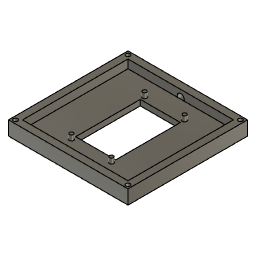
case top (Autodesk Fusion 360 design; units mm, degrees)
Autodesk Fusion 360 part; units mm, degrees
note: some values were not read from the file. Set by a fixed rule: which sketch regions a step uses.
sketch "Sketch1" plane through (0, 0, 0) normal (0, 0, 1) x (1, 0, 0)
  line L0 (0, 0) -> (0, 75)
  line L1 (0, 75) -> (75, 75)
  line L2 (0, 0) -> (75, 0)
  line L3 (75, 0) -> (75, 75)
  line L4 (75, 75) -> (0, 75)
  line L5 (0, 75) -> (0, 0)
  line L6 (-5, -5) -> (80, -5)
  line L7 (80, -5) -> (80, 80)
  line L8 (80, 80) -> (-5, 80)
  line L9 (-5, 80) -> (-5, -5)
  line L10 (-5, -5) -> (80, -5)
  line L11 (80, -5) -> (80, 80)
  dimension "d1" = 75
  dimension "d2" = 75
  dimension "d3" = 85
  constraint coincident L0.start L2.start
  constraint vertical L0
  constraint perpendicular L0 L1
  constraint horizontal L2
  constraint vertical L3
  constraint horizontal L4
  constraint vertical L5
  constraint horizontal L6
  constraint perpendicular L6 L7
  constraint horizontal L8
  constraint vertical L9
  constraint horizontal L10
  constraint vertical L11
  measures "d1" distance of L0.start L0.end
  measures "d2" distance of L0.end L1.end
  measures "d3" distance of L6.end L7.end
extrude "Extrude1" add sketch "Sketch1" along normal blind 10
sketch "Sketch2" plane through (0, 0, 0) normal (0, 0, 1) x (1, 0, 0)
  line L0 (0, 0) -> (75, 0)
  line L1 (75, 0) -> (75, 75)
  line L2 (75, 75) -> (0, 75)
  line L3 (0, 75) -> (0, 0)
  constraint horizontal L0
  constraint vertical L1
  constraint horizontal L2
  constraint vertical L3
  constraint coincident L0.start L3.end
extrude "Extrude2" add sketch "Sketch2" along normal blind 4
sketch "Sketch3" plane through (0, 0, 4) normal (0, 0, 1) x (-1, 0, 0)
  line L0 (0, -75) -> (0, 0)
  line L1 (0, 0) -> (-75, 0)
  line L2 (-75, 0) -> (-75, -75)
  line L3 (-75, -75) -> (0, -75)
  line L4 (0, -75) -> (-75, 0)
  line L5 (0, 0) -> (-75, -75)
  line L6 (-37.5, -37.5) -> (-20.25, -37.5)
  line L7 (-37.5, -37.5) -> (-54.75, -37.5)
  line L8 (-20.25, -37.5) -> (-20.25, -66.5)
  line L9 (-54.75, -37.5) -> (-54.75, -8.5)
  line L10 (-20.25, -66.5) -> (-54.75, -66.5)
  line L11 (-54.75, -66.5) -> (-54.75, -8.5)
  line L12 (-54.75, -8.5) -> (-20.25, -8.5)
  line L13 (-20.25, -8.5) -> (-20.25, -66.5)
  line L14 (-37.5, -37.5) -> (-37.5, -60.5)
  line L15 (-37.5, -37.5) -> (-37.5, -14.5)
  line L16 (-37.5, -14.5) -> (-51.75, -14.5)
  line L17 (-37.5, -60.5) -> (-23.25, -60.5)
  line L18 (-23.25, -60.5) -> (-51.75, -60.5)
  line L19 (-51.75, -60.5) -> (-51.75, -14.5)
  line L20 (-51.75, -14.5) -> (-23.25, -14.5)
  line L21 (-23.25, -14.5) -> (-23.25, -60.5)
  dimension "d8" = 17.25
  dimension "d9" = 17.25
  dimension "d10" = 29
  dimension "d11" = 29
  dimension "d12" = 23
  dimension "d13" = 23
  dimension "d14" = 14.25
  dimension "d15" = 14.25
  constraint coincident L0.start L3.end
  constraint coincident L1.end L2.start
  constraint coincident L0.end L1.start
  constraint coincident L2.end L3.start
  constraint midpoint L4 L6.start
  constraint parallel L3 L6
  constraint parallel L6 L7
  constraint perpendicular L6 L8
  constraint perpendicular L7 L9
  constraint horizontal L10
  constraint vertical L11
  constraint horizontal L12
  constraint vertical L13
  constraint perpendicular L6 L14
  constraint perpendicular L7 L15
  constraint perpendicular L15 L16
  constraint perpendicular L14 L17
  constraint horizontal L18
  constraint vertical L19
  constraint horizontal L20
  constraint vertical L21
  measures "d8" distance of L6.start L6.end
  measures "d9" distance of L6.start L7.end
  measures "d10" distance of L6.end L8.end
  measures "d11" distance of L7.end L9.end
  measures "d12" distance of L6.start L14.end
  measures "d13" distance of L6.start L15.end
  measures "d14" distance of L15.end L16.end
  measures "d15" distance of L14.end L17.end
extrude "Extrude3" cut sketch "Sketch3" against normal blind 5 contours L4 L14 L17 L18 L21 | L4 L6 L21 | L5 L6 L21 | L5 L15 L20 L21 | L5 L7 L19 | L5 L14 L18 L19 | L4 L7 L19 | L4 L15 L16 L19 L20
sketch "Sketch4" plane through (0, 0, 4) normal (0, 0, 1) x (-1, 0, 0)
  line L0 (-51.75, -60.5) -> (-51.75, -14.5)
  line L1 (-51.75, -14.5) -> (-23.25, -14.5)
  line L2 (-23.25, -14.5) -> (-23.25, -60.5)
  line L3 (-23.25, -60.5) -> (-51.75, -60.5)
  line L4 (0, -75) -> (0, 0)
  line L5 (0, 0) -> (-75, 0)
  line L6 (-75, 0) -> (-75, -75)
  line L7 (-75, -75) -> (0, -75)
  line L8 (-75, 0) -> (0, -75)
  line L9 (-75, -75) -> (0, 0)
  line L10 (-37.5, -37.5) -> (-54.75, -37.5)
  line L11 (-54.75, -37.5) -> (-54.75, -8.5)
  line L12 (-54.75, -8.5) -> (-20.25, -8.5)
  line L13 (-20.25, -8.5) -> (-20.25, -66.5)
  line L14 (-20.25, -66.5) -> (-54.75, -66.5)
  line L15 (-54.75, -66.5) -> (-54.75, -8.5)
  line L16 (-54.75, -8.5) -> (-20.25, -8.5)
  line L17 (-20.25, -8.5) -> (-20.25, -66.5)
  line L18 (-20.25, -66.5) -> (-20.25, -63.5)
  line L19 (-20.25, -63.5) -> (-23.25, -63.5)
  circle A0 centre (-23.25, -63.5) radius 1.6
  line L20 (-54.75, -66.5) -> (-51.75, -66.5)
  line L21 (-51.75, -66.5) -> (-51.75, -63.5)
  circle A1 centre (-51.75, -63.5) radius 1.6
  line L22 (-20.25, -8.5) -> (-23.25, -8.5)
  line L23 (-23.25, -8.5) -> (-23.25, -11.5)
  circle A2 centre (-23.25, -11.5) radius 1.6
  line L24 (-54.75, -8.5) -> (-54.75, -11.5)
  line L25 (-54.75, -11.5) -> (-51.75, -11.5)
  circle A3 centre (-51.75, -11.5) radius 1.6
  dimension "d23" = 17.25
  dimension "d24" = 29
  dimension "d25" = 34.5
  dimension "d26" = 58
  dimension "d27" = 3
  dimension "d28" = 3
  dimension "d29" = 3.2
  dimension "d30" = 3
  dimension "d31" = 3
  dimension "d32" = 3.2
  dimension "d33" = 3
  dimension "d34" = 3
  dimension "d35" = 3.2
  dimension "d36" = 3
  dimension "d37" = 3
  dimension "d38" = 3.2
  constraint coincident L5.end L6.start
  constraint coincident L4.start L7.end
  constraint coincident L6.end L7.start
  constraint coincident L4.end L5.start
  constraint midpoint L8 L10.start
  constraint parallel L5 L10
  constraint perpendicular L10 L11
  constraint perpendicular L11 L12
  constraint perpendicular L1 L13
  constraint horizontal L14
  constraint vertical L15
  constraint horizontal L16
  constraint vertical L17
  constraint perpendicular L14 L18
  constraint perpendicular L17 L19
  constraint coincident L19.end A0.centre
  constraint perpendicular L15 L20
  constraint perpendicular L20 L21
  constraint coincident L21.end A1.centre
  constraint perpendicular L17 L22
  constraint perpendicular L12 L23
  constraint coincident L23.end A2.centre
  constraint perpendicular L12 L24
  constraint perpendicular L24 L25
  constraint coincident L25.end A3.centre
  measures "d23" distance of L10.start L10.end
  measures "d24" distance of L10.end L11.end
  measures "d25" distance of L11.end L12.end
  measures "d26" distance of L12.end L13.end
  measures "d27" distance of L13.end L18.end
  measures "d28" distance of L18.end L19.end
  measures "d29" diameter of A0
  measures "d30" distance of L14.end L20.end
  measures "d31" distance of L20.end L21.end
  measures "d32" diameter of A1
  measures "d33" distance of L12.end L22.end
  measures "d34" distance of L22.end L23.end
  measures "d35" diameter of A2
  measures "d36" distance of L11.end L24.end
  measures "d37" distance of L24.end L25.end
  measures "d38" diameter of A3
extrude "Extrude4" add sketch "Sketch4" along normal blind 3.5 draft -4 contours A0 | A1 | A2 | A3
sketch "Sketch5" plane through (0, 0, 10) normal (0, 0, 1) x (-1, 0, 0)
  line L0 (0, 0) -> (0, -75)
  line L1 (0, -75) -> (-75, -75)
  line L2 (-75, -75) -> (-75, 0)
  line L3 (-75, 0) -> (0, 0)
  line L4 (-80, 5) -> (-80, -80)
  line L5 (-80, -80) -> (5, -80)
  line L6 (5, -80) -> (5, 5)
  line L7 (5, 5) -> (-80, 5)
  line L8 (5, 5) -> (0, 0)
  line L9 (5, 0) -> (0, 5)
  circle A0 centre (2.5, 2.5) radius 1.5
  line L10 (-75, 0) -> (-80, 5)
  circle A1 centre (-77.5, 2.5) radius 1.5
  line L11 (-75, 5) -> (-80, 0)
  circle A2 centre (-77.5, -77.5) radius 1.5
  circle A3 centre (2.5, -77.5) radius 1.5
  dimension "d41" = 3
  dimension "d43" = 3
  dimension "d44" = 3
  dimension "d45" = 3
  constraint coincident L6.end L7.start
  constraint coincident L0.start L3.end
  constraint coincident L6 L9.start
  constraint perpendicular L8 L9
  constraint midpoint L8 A0.centre
  constraint coincident L2.end L3.start
  constraint coincident L4.start L7.end
  constraint midpoint L10 A1.centre
  constraint coincident L7 L11.start
  constraint coincident L4 L11.end
  measures "d41" diameter of A0
  measures "d43" diameter of A1
  measures "d44" diameter of A2
  measures "d45" diameter of A3
extrude "Extrude5" cut sketch "Sketch5" against normal blind 4 contours L8 L9 A0 | L8 L9 A0 | L10 A1 L11 | L10 A1 L11 | L8 L9 A0 | L8 L9 A0 | L10 A1 L11 | L10 A1 L11 | A2 | A3
sketch "Sketch6" plane through (0, 75, 0) normal (0, -1, 0) x (1, 0, 0)
  line L0 (0, 4) -> (75, 4)
  line L1 (75, 4) -> (75, 10)
  line L2 (75, 10) -> (0, 10)
  line L3 (0, 10) -> (0, 4)
  line L4 (75, 4) -> (0, 10)
  line L5 (0, 4) -> (75, 10)
  line L6 (38.5, 6.7) -> (36.5, 6.7)
  line L7 (36.5, 6.7) -> (36.5, 7.3)
  line L8 (36.5, 7.3) -> (38.5, 7.3)
  line L9 (38.5, 7.3) -> (38.5, 6.7)
  line L10 (38.5, 6.7) -> (36.5, 7.3) construction
  line L11 (36.5, 6.7) -> (38.5, 7.3) construction
  point P0 (37.5, 7)
  constraint coincident L0.end L1.start
  constraint coincident L2.end L3.start
  constraint coincident L0.start L3.end
  constraint coincident L1.end L2.start
  constraint horizontal L6
  constraint perpendicular L6 L7
  constraint parallel L6 L8
  constraint parallel L7 L9
  constraint coincident L10 P0
  constraint coincident L11 P0
  constraint midpoint L4 P0
extrude "Extrude6" cut sketch "Sketch6" against normal blind 5 contours L4 L5 L7 | L4 L5 L6 L7 L9 | L4 L5 L9 | L4 L5 L7 L8 L9
sketch "Sketch7" plane through (0, 80, 0) normal (0, 1, 0) x (-1, 0, 0)
  line L0 (-36.5, 7.3) -> (-36.5, 6.7)
  line L1 (-38.5, 6.7) -> (-38.5, 7.3)
  line L2 (-80, 0) -> (5, 0)
  line L3 (5, 0) -> (5, 10)
  line L4 (5, 10) -> (-80, 10)
  line L5 (-80, 10) -> (-80, 0)
  line L6 (5, 0) -> (-80, 10)
  line L7 (-80, 0) -> (5, 10)
  circle A0 centre (-37.5, 5) radius 2.5
  dimension "d50" = 5
  constraint coincident L2.end L3.start
  constraint coincident L4.end L5.start
  constraint coincident L2.start L5.end
  constraint coincident L3.end L4.start
  constraint midpoint L6 A0.centre
  measures "d50" diameter of A0
extrude "Extrude7" cut sketch "Sketch7" against normal blind 5 contours L6 L7 A0 | L6 L7 A0 | L6 L7 A0 | L6 L7 A0
equation "d8 = ( 34.5 / 2 ) * 1 mm"
equation "d9 = ( 34.5 / 2 ) * 1 mm"
equation "d10 = ( 58 / 2 ) * 1 mm"
equation "d11 = ( 58 / 2 ) * 1 mm"
equation "d12 = ( 46 / 2 ) * 1 mm"
equation "d13 = ( 46 / 2 ) * 1 mm"
equation "d14 = ( 28.5 / 2 ) * 1 mm"
equation "d15 = ( 28.5 / 2 ) * 1 mm"
equation "d23 = ( 34.5 / 2 ) * 1 mm"
equation "d24 = ( 58 / 2 ) * 1 mm"
